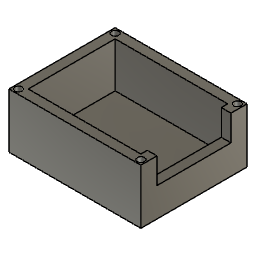
Bottom Battery Holder v2 (Autodesk Fusion 360 design; units mm, degrees)
Autodesk Fusion 360 part; units mm, degrees
(part 1 of 2)
sketch "Sketch1" plane through (0, 0, 0) normal (0, 0, 1) x (1, 0, 0)
  line L0 (0, 0) -> (41, 0)
  line L1 (41, 0) -> (41, 33)
  line L2 (41, 33) -> (0, 33)
  line L3 (0, 33) -> (0, 0)
  dimension "d1" = 41
  dimension "d2" = 33
  constraint horizontal L0
  constraint vertical L1
  constraint horizontal L2
  constraint vertical L3
  constraint coincident L0.start L3.end
  measures "d1" distance of L0.start L0.end
  measures "d2" distance of L0.start L2.end
extrude "Extrude1" add sketch "Sketch1" along normal blind 17
sketch "Sketch2" plane through (0, 0, 17) normal (0, 0, 1) x (-1, 0, 0)
  line L0 (0, -33) -> (0, 0)
  line L1 (0, 0) -> (-41, 0)
  line L2 (-41, 0) -> (-41, -33)
  line L3 (-41, -33) -> (0, -33)
  line L4 (-3, -3) -> (-38, -3)
  line L5 (-38, -3) -> (-38, -30)
  line L6 (-38, -30) -> (-3, -30)
  line L7 (-3, -30) -> (-3, -3)
  dimension "d5" = 35
  dimension "d6" = 27
  constraint horizontal L4
  constraint vertical L5
  constraint horizontal L6
  constraint vertical L7
  measures "d5" distance of L4.start L4.end
  measures "d6" distance of L4.start L6.end
extrude "Extrude2" cut sketch "Sketch2" against normal blind 14 contours L4 L5 L6 L7
sketch "Sketch3" plane through (41, 0, 0) normal (1, 0, 0) x (0, 1, 0)
  line L0 (0, 0) -> (33, 0)
  line L1 (33, 0) -> (33, 17)
  line L2 (33, 17) -> (0, 17)
  line L3 (0, 17) -> (0, 0)
  line L4 (4.9994, 17) -> (28, 17)
  line L5 (28, 17) -> (28, 9)
  line L6 (28, 9) -> (4.9994, 9)
  line L7 (4.9994, 9) -> (4.9994, 17)
  constraint horizontal L4
  constraint vertical L5
  constraint horizontal L6
  constraint vertical L7
  constraint coincident L2 L4.start
extrude "Extrude3" cut sketch "Sketch3" against normal blind 10 contours L2 L4 L5 L6 L7
sketch "Sketch4" plane through (0, 0, 17) normal (0, 0, 1) x (-1, 0, 0)
  line L0 (-41, -4.9994) -> (-38, -4.9994)
  line L1 (-38, -4.9994) -> (-38, -3)
  line L2 (-38, -3) -> (-3, -3)
  line L3 (-3, -3) -> (-3, -30)
  line L4 (-3, -30) -> (-38, -30)
  line L5 (-38, -30) -> (-38, -28)
  line L6 (-38, -28) -> (-41, -28)
  line L7 (-41, -28) -> (-41, -33)
  line L8 (-41, -33) -> (0, -33)
  line L9 (0, -33) -> (0, 0)
  line L10 (0, 0) -> (-41, 0)
  line L11 (-41, 0) -> (-41, -4.9994)
  circle A0 centre (-1.5, -31.5) radius 1.118
  circle A1 centre (-1.5, -1.4974) radius 1.1192
  circle A2 centre (-39.5, -1.5) radius 1.118
  circle A3 centre (-39.5, -31.5) radius 1.118
  dimension "d11" = 2.2384
  dimension "d12" = 2.2361
  dimension "d13" = 2.236
  measures "d11" diameter of A1
  measures "d12" diameter of A0
  measures "d13" diameter of A3
extrude "Extrude4" cut sketch "Sketch4" against normal blind 10 contours A0 | A1 | A2 | A3
sketch "falmouthrobotics" plane through (0, 0, 0) normal (0, 0, -1) x (-1, 0, 0)
  arc A0 through (-5.6563, 11.59, -1.2301) (-5.3945, 11.4792, -1.2301) (-5.1327, 11.3684, -1.2301)
  arc A1 through (-5.1327, 11.3684, -1.2301) (-5.117, 11.3607, -1.2301) (-5.1022, 11.3515, -1.2301)
  arc A2 through (-32.1117, 13.7154, -1.2301) (-32.0879, 13.6563, -1.2301) (-32.0476, 13.607, -1.2301)
  arc A3 through (-15.3811, 14.3738, -1.2301) (-15.4462, 14.3529, -1.2301) (-15.5092, 14.3263, -1.2301)
  line L0 (-34.3881, 15.5149, -1.2301) -> (-33.2917, 15.5149, -1.2301)
  arc A4 through (-8.6784, 13.2928, -1.2301) (-8.7193, 13.2009, -1.2301) (-8.7575, 13.1079, -1.2301)
  arc A5 through (-7.6435, 12.4319, -1.2301) (-7.2917, 12.278, -1.2301) (-6.9381, 12.1281, -1.2301)
  arc A6 through (-5.1022, 11.3515, -1.2301) (-5.0953, 11.3416, -1.2301) (-5.0965, 11.3296, -1.2301)
  arc A7 through (-5.1403, 11.2447, -1.2301) (-5.1702, 11.1924, -1.2301) (-5.2021, 11.1412, -1.2301)
  arc A8 through (-15.5881, 14.2649, -1.2301) (-15.6327, 14.1862, -1.2301) (-15.6472, 14.0969, -1.2301)
  line L1 (-34.3881, 14.6527, -1.2301) -> (-34.3881, 15.5149, -1.2301)
  arc A9 through (-33.2653, 15.9925, -1.2301) (-33.6488, 15.998, -1.2301) (-34.0323, 16.0007, -1.2301)
  line L2 (-32.1954, 15.5149, -1.2301) -> (-32.1667, 14.5399, -1.2301)
  arc A10 through (-14.5007, 14.281, -1.2301) (-14.6017, 14.3449, -1.2301) (-14.7151, 14.3826, -1.2301)
  arc A11 through (-6.2455, 11.8382, -1.2301) (-5.9508, 11.7143, -1.2301) (-5.6563, 11.59, -1.2301)
  arc A12 through (-8.7575, 13.1079, -1.2301) (-8.7675, 13.0656, -1.2301) (-8.7654, 13.0223, -1.2301)
  arc A13 through (-32.1444, 13.9508, -1.2301) (-32.1335, 13.8323, -1.2301) (-32.1117, 13.7154, -1.2301)
  line L3 (-32.7772, 12.1034, -1.2301) -> (-34.3881, 13.7905, -1.2301)
  arc A14 through (-4.5188, 11.422, -1.2301) (-4.5087, 11.4642, -1.2301) (-4.5108, 11.5076, -1.2301)
  line L4 (-6.7536, 14.2928, -1.2301) -> (-8.0692, 14.3206, -1.2301)
  line L5 (-7.9945, 13.506, -1.2301) -> (-7.779, 13.8087, -1.2301)
  arc A15 through (-8.7654, 13.0223, -1.2301) (-8.745, 12.9761, -1.2301) (-8.7064, 12.9436, -1.2301)
  arc A16 through (-8.5827, 10.2892, -1.2301) (-8.3781, 10.2689, -1.2301) (-8.1726, 10.2591, -1.2301)
  line L6 (-30.4381, 10.1649, -1.2301) -> (-28.9381, 10.1649, -1.2301)
  arc A17 through (-4.5977, 11.2373, -1.2301) (-4.5568, 11.329, -1.2301) (-4.5188, 11.422, -1.2301)
  line L7 (-28.9381, 10.1649, -1.2301) -> (-27.4381, 10.1649, -1.2301)
  arc A18 through (-5.4381, 14.0649, -1.2301) (-5.4521, 14.1267, -1.2301) (-5.4914, 14.1764, -1.2301)
  arc A19 through (-14.7151, 14.3826, -1.2301) (-14.8758, 14.4068, -1.2301) (-15.0381, 14.4149, -1.2301)
  arc A20 through (-8.1361, 13.2849, -1.2301) (-8.1062, 13.3371, -1.2301) (-8.0745, 13.3882, -1.2301)
  line L8 (-34.3381, 13.0329, -1.2301) -> (-32.9548, 11.5739, -1.2301)
  arc A21 through (-28.9152, 14.0926, -1.2301) (-29.2888, 14.0982, -1.2301) (-29.6625, 14.1009, -1.2301)
  arc A22 through (-8.1436, 13.1615, -1.2301) (-8.1592, 13.1691, -1.2301) (-8.174, 13.1783, -1.2301)
  arc A23 through (-29.6625, 14.1009, -1.2301) (-29.8782, 14.0978, -1.2301) (-30.0937, 14.0871, -1.2301)
  arc A24 through (-8.601, 10.6404, -1.2301) (-8.691, 10.6185, -1.2301) (-8.7746, 10.5784, -1.2301)
  arc A25 through (-7.0308, 12.6917, -1.2301) (-7.3254, 12.8156, -1.2301) (-7.6199, 12.9399, -1.2301)
  arc A26 through (-31.9381, 13.5649, -1.2301) (-31.8778, 13.5777, -1.2301) (-31.828, 13.614, -1.2301)
  arc A27 through (-7.1682, 10.6923, -1.2301) (-7.6947, 10.6826, -1.2301) (-8.2211, 10.6708, -1.2301)
  line L9 (-31.7381, 14.7649, -1.2301) -> (-31.7381, 15.9649, -1.2301)
  arc A28 through (-31.5196, 10.1515, -1.2301) (-31.4766, 10.1244, -1.2301) (-31.4267, 10.1149, -1.2301)
  arc A29 through (-15.5756, 13.9489, -1.2301) (-15.4746, 13.885, -1.2301) (-15.3612, 13.8472, -1.2301)
  arc A30 through (-8.7064, 12.9436, -1.2301) (-8.4675, 12.8229, -1.2301) (-8.2277, 12.7043, -1.2301)
  arc A31 through (-5.0965, 11.3296, -1.2301) (-5.1179, 11.2869, -1.2301) (-5.1403, 11.2447, -1.2301)
  arc A32 through (-34.7609, 15.9565, -1.2301) (-34.8102, 15.9347, -1.2301) (-34.8419, 15.8912, -1.2301)
  arc A33 through (-31.7673, 13.7399, -1.2301) (-31.7496, 13.8786, -1.2301) (-31.7426, 14.0182, -1.2301)
  line L10 (-31.7381, 15.9649, -1.2301) -> (-33.2653, 15.9925, -1.2301)
  arc A34 through (-15.5092, 14.3263, -1.2301) (-15.552, 14.2999, -1.2301) (-15.5881, 14.2649, -1.2301)
  arc A35 through (-5.2021, 11.1412, -1.2301) (-5.2415, 11.0817, -1.2301) (-5.2823, 11.0231, -1.2301)
  arc A36 through (-34.0323, 16.0007, -1.2301) (-34.2562, 15.9976, -1.2301) (-34.4798, 15.987, -1.2301)
  arc A37 through (-8.5675, 13.511, -1.2301) (-8.6249, 13.4029, -1.2301) (-8.6784, 13.2928, -1.2301)
  line L11 (-34.3881, 13.7905, -1.2301) -> (-34.3881, 14.6527, -1.2301)
  line L12 (-5.2823, 11.0231, -1.2301) -> (-5.4983, 10.7197, -1.2301)
  arc A38 through (-15.6472, 14.0969, -1.2301) (-15.6277, 14.015, -1.2301) (-15.5756, 13.9489, -1.2301)
  arc A39 through (-8.2277, 12.7043, -1.2301) (-7.9369, 12.5653, -1.2301) (-7.6435, 12.4319, -1.2301)
  arc A40 through (-32.1667, 14.5399, -1.2301) (-32.1568, 14.2453, -1.2301) (-32.1444, 13.9508, -1.2301)
  line L13 (-5.4983, 10.7197, -1.2301) -> (-7.1682, 10.6923, -1.2301)
  arc A41 through (-31.9353, 10.5435, -1.2301) (-31.7281, 10.3469, -1.2301) (-31.5196, 10.1515, -1.2301)
  arc A42 through (-31.2884, 10.2421, -1.2301) (-31.3002, 10.3789, -1.2301) (-31.357, 10.5039, -1.2301)
  arc A43 through (-31.828, 13.614, -1.2301) (-31.7886, 13.6726, -1.2301) (-31.7673, 13.7399, -1.2301)
  arc A44 through (-14.4881, 13.9649, -1.2301) (-14.4435, 14.0437, -1.2301) (-14.429, 14.133, -1.2301)
  arc A45 through (-8.4309, 13.7428, -1.2301) (-8.5008, 13.6278, -1.2301) (-8.5675, 13.511, -1.2301)
  arc A46 through (-31.4267, 10.1149, -1.2301) (-31.3327, 10.1516, -1.2301) (-31.2884, 10.2421, -1.2301)
  arc A47 through (-15.0381, 13.8149, -1.2301) (-14.947, 13.8175, -1.2301) (-14.8563, 13.8252, -1.2301)
  arc A48 through (-32.0476, 13.607, -1.2301) (-31.9968, 13.5758, -1.2301) (-31.9381, 13.5649, -1.2301)
  arc A49 through (-30.4723, 12.7289, -1.2301) (-30.4698, 12.3703, -1.2301) (-30.4655, 12.0117, -1.2301)
  line L14 (-33.2917, 15.5149, -1.2301) -> (-32.1954, 15.5149, -1.2301)
  arc A50 through (-32.4141, 11.0147, -1.2301) (-32.1765, 10.7773, -1.2301) (-31.9353, 10.5435, -1.2301)
  arc A51 through (-5.0486, 11.8256, -1.2301) (-5.3394, 11.9645, -1.2301) (-5.6327, 12.098, -1.2301)
  arc A52 through (-7.6199, 12.9399, -1.2301) (-7.8818, 13.0507, -1.2301) (-8.1436, 13.1615, -1.2301)
  arc A53 through (-4.8449, 10.7877, -1.2301) (-4.7752, 10.9025, -1.2301) (-4.7085, 11.0192, -1.2301)
  arc A54 through (-30.47, 13.3545, -1.2301) (-30.4724, 13.0417, -1.2301) (-30.4723, 12.7289, -1.2301)
  arc A55 through (-5.4914, 14.1764, -1.2301) (-5.5572, 14.217, -1.2301) (-5.631, 14.2397, -1.2301)
  line L15 (-27.4381, 14.0649, -1.2301) -> (-28.9152, 14.0926, -1.2301)
  line L16 (-5.2063, 10.2105, -1.2301) -> (-4.8449, 10.7877, -1.2301)
  arc A56 through (-4.5108, 11.5076, -1.2301) (-4.5313, 11.5538, -1.2301) (-4.5699, 11.5863, -1.2301)
  arc A57 through (-4.7085, 11.0192, -1.2301) (-4.6512, 11.1272, -1.2301) (-4.5977, 11.2373, -1.2301)
  arc A58 through (-5.6327, 12.098, -1.2301) (-5.9846, 12.2518, -1.2301) (-6.3381, 12.4017, -1.2301)
  arc A59 through (-8.0745, 13.3882, -1.2301) (-8.0351, 13.4476, -1.2301) (-7.9945, 13.506, -1.2301)
  line L17 (-7.779, 13.8087, -1.2301) -> (-6.6085, 13.8368, -1.2301)
  line L18 (-8.0692, 14.3206, -1.2301) -> (-8.4309, 13.7428, -1.2301)
  arc A60 through (-8.7746, 10.5784, -1.2301) (-8.8212, 10.53, -1.2301) (-8.8381, 10.4649, -1.2301)
  arc A61 through (-5.631, 14.2397, -1.2301) (-5.7836, 14.2607, -1.2301) (-5.9373, 14.271, -1.2301)
  arc A62 through (-5.9373, 14.271, -1.2301) (-6.3454, 14.283, -1.2301) (-6.7536, 14.2928, -1.2301)
  arc A63 through (-8.8381, 10.4649, -1.2301) (-8.8201, 10.3986, -1.2301) (-8.7708, 10.3506, -1.2301)
  line L19 (-27.4381, 10.1649, -1.2301) -> (-27.4381, 12.1149, -1.2301)
  arc A64 through (-8.174, 13.1783, -1.2301) (-8.1809, 13.1882, -1.2301) (-8.1798, 13.2002, -1.2301)
  arc A65 through (-8.1726, 10.2591, -1.2301) (-7.5974, 10.2474, -1.2301) (-7.0222, 10.2377, -1.2301)
  line L20 (-30.4655, 12.0117, -1.2301) -> (-30.4381, 10.1649, -1.2301)
  arc A66 through (-5.4868, 13.9542, -1.2301) (-5.4508, 14.0045, -1.2301) (-5.4381, 14.0649, -1.2301)
  arc A67 through (-8.1798, 13.2002, -1.2301) (-8.1585, 13.2429, -1.2301) (-8.1361, 13.2849, -1.2301)
  arc A68 through (-30.4621, 13.8893, -1.2301) (-30.4665, 13.6219, -1.2301) (-30.47, 13.3545, -1.2301)
  arc A69 through (-4.5699, 11.5863, -1.2301) (-4.8087, 11.7069, -1.2301) (-5.0486, 11.8256, -1.2301)
  line L21 (-27.4381, 12.1149, -1.2301) -> (-27.4381, 14.0649, -1.2301)
  arc A70 through (-8.7708, 10.3506, -1.2301) (-8.6797, 10.3109, -1.2301) (-8.5827, 10.2892, -1.2301)
  arc A71 through (-6.3381, 12.4017, -1.2301) (-6.6845, 12.5466, -1.2301) (-7.0308, 12.6917, -1.2301)
  line L22 (-7.0222, 10.2377, -1.2301) -> (-5.2063, 10.2105, -1.2301)
  arc A72 through (-6.6085, 13.8368, -1.2301) (-6.2487, 13.8466, -1.2301) (-5.889, 13.8588, -1.2301)
  arc A73 through (-5.889, 13.8588, -1.2301) (-5.7504, 13.8693, -1.2301) (-5.6129, 13.8906, -1.2301)
  arc A74 through (-30.4426, 13.9894, -1.2301) (-30.4567, 13.9402, -1.2301) (-30.4621, 13.8893, -1.2301)
  arc A75 through (-8.2211, 10.6708, -1.2301) (-8.4115, 10.6609, -1.2301) (-8.601, 10.6404, -1.2301)
  arc A76 through (-5.6129, 13.8906, -1.2301) (-5.5455, 13.9137, -1.2301) (-5.4868, 13.9542, -1.2301)
  arc A77 through (-22.3721, 21.0063, -1.2301) (-22.5314, 21.0347, -1.2301) (-22.6925, 21.0501, -1.2301)
  arc A78 through (-20.2423, 17.2748, -1.2301) (-20.1749, 17.3588, -1.2301) (-20.1417, 17.4613, -1.2301)
  arc A79 through (-20.123, 17.9253, -1.2301) (-20.1529, 18.4515, -1.2301) (-20.1882, 18.9774, -1.2301)
  arc A80 through (-20.8687, 20.3549, -1.2301) (-20.7876, 20.1081, -1.2301) (-20.7457, 19.8517, -1.2301)
  arc A81 through (-31.3022, 19.6901, -1.2301) (-31.4368, 19.2445, -1.2301) (-31.5647, 18.7969, -1.2301)
  arc A82 through (-31.1005, 17.5695, -1.2301) (-30.9592, 17.5368, -1.2301) (-30.8157, 17.515, -1.2301)
  arc A83 through (-29.6034, 17.4414, -1.2301) (-29.4771, 17.4467, -1.2301) (-29.3512, 17.4562, -1.2301)
  arc A84 through (-23.9816, 21.4831, -1.2301) (-24.047, 21.5096, -1.2301) (-24.1176, 21.5076, -1.2301)
  line L23 (-30.5878, 20.6825, -1.2301) -> (-31.0375, 20.543, -1.2301)
  arc A85 through (-20.7284, 20.9621, -1.2301) (-20.847, 21.0193, -1.2301) (-20.974, 21.054, -1.2301)
  arc A86 through (-30.3134, 17.4669, -1.2301) (-30.1203, 17.4535, -1.2301) (-29.9269, 17.4438, -1.2301)
  arc A87 through (-28.7881, 20.9358, -1.2301) (-28.7899, 20.8267, -1.2301) (-28.7952, 20.7177, -1.2301)
  arc A88 through (-20.974, 21.054, -1.2301) (-21.1103, 21.0662, -1.2301) (-21.2466, 21.0547, -1.2301)
  arc A89 through (-24.1176, 21.5076, -1.2301) (-24.183, 21.4775, -1.2301) (-24.232, 21.4248, -1.2301)
  arc A90 through (-23.7217, 20.819, -1.2301) (-23.7327, 20.8159, -1.2301) (-23.744, 20.8149, -1.2301)
  arc A91 through (-20.4913, 17.3172, -1.2301) (-20.4631, 17.2726, -1.2301) (-20.4189, 17.2437, -1.2301)
  arc A92 through (-28.7832, 21.0731, -1.2301) (-28.7869, 21.0045, -1.2301) (-28.7881, 20.9358, -1.2301)
  arc A93 through (-20.5898, 17.8097, -1.2301) (-20.5714, 17.6585, -1.2301) (-20.5452, 17.5083, -1.2301)
  arc A94 through (-28.7952, 20.7177, -1.2301) (-28.806, 20.6779, -1.2301) (-28.8315, 20.6455, -1.2301)
  arc A95 through (-30.2665, 20.7566, -1.2301) (-30.4285, 20.7255, -1.2301) (-30.5878, 20.6825, -1.2301)
  arc A96 through (-29.9269, 17.4438, -1.2301) (-29.7652, 17.4399, -1.2301) (-29.6034, 17.4414, -1.2301)
  arc A97 through (-23.7754, 20.9102, -1.2301) (-23.7847, 20.9624, -1.2301) (-23.7925, 21.0148, -1.2301)
  arc A98 through (-20.7457, 19.8517, -1.2301) (-20.6831, 19.0671, -1.2301) (-20.6278, 18.282, -1.2301)
  arc A99 through (-23.7925, 21.0148, -1.2301) (-23.8002, 21.0769, -1.2301) (-23.8068, 21.1391, -1.2301)
  arc A100 through (-21.5495, 20.9666, -1.2301) (-21.6891, 20.9127, -1.2301) (-21.8313, 20.8664, -1.2301)
  arc A101 through (-23.3635, 20.9608, -1.2301) (-23.4314, 20.9326, -1.2301) (-23.4995, 20.9049, -1.2301)
  arc A102 through (-22.07, 20.8212, -1.2301) (-22.1517, 20.8204, -1.2301) (-22.2326, 20.8323, -1.2301)
  arc A103 through (-28.7215, 21.3483, -1.2301) (-28.7375, 21.3271, -1.2301) (-28.7474, 21.3024, -1.2301)
  arc A104 through (-20.4189, 17.2437, -1.2301) (-20.3263, 17.2348, -1.2301) (-20.2423, 17.2748, -1.2301)
  arc A105 through (-31.6486, 18.3294, -1.2301) (-31.6462, 18.176, -1.2301) (-31.6134, 18.0261, -1.2301)
  arc A106 through (-23.7576, 20.8258, -1.2301) (-23.7669, 20.8679, -1.2301) (-23.7754, 20.9102, -1.2301)
  arc A107 through (-23.8068, 21.1391, -1.2301) (-23.8262, 21.2445, -1.2301) (-23.8633, 21.3451, -1.2301)
  arc A108 through (-28.7474, 21.3024, -1.2301) (-28.7591, 21.2512, -1.2301) (-28.7685, 21.1996, -1.2301)
  arc A109 through (-31.4628, 17.7805, -1.2301) (-31.383, 17.7104, -1.2301) (-31.2949, 17.6511, -1.2301)
  arc A110 through (-23.0627, 21.0391, -1.2301) (-23.2159, 21.0106, -1.2301) (-23.3635, 20.9608, -1.2301)
  arc A111 through (-22.2881, 20.9018, -1.2301) (-22.3117, 20.9689, -1.2301) (-22.3721, 21.0063, -1.2301)
  arc A112 through (-22.6925, 21.0501, -1.2301) (-22.8778, 21.0524, -1.2301) (-23.0627, 21.0391, -1.2301)
  arc A113 through (-21.1031, 20.5148, -1.2301) (-20.9622, 20.4696, -1.2301) (-20.8687, 20.3549, -1.2301)
  line L24 (-31.0375, 20.543, -1.2301) -> (-31.3022, 19.6901, -1.2301)
  arc A114 through (-20.6278, 18.282, -1.2301) (-20.6105, 18.0457, -1.2301) (-20.5898, 17.8097, -1.2301)
  arc A115 through (-28.8315, 20.6455, -1.2301) (-28.8672, 20.6264, -1.2301) (-28.9076, 20.6235, -1.2301)
  arc A116 through (-23.4995, 20.9049, -1.2301) (-23.5593, 20.8811, -1.2301) (-23.6192, 20.8578, -1.2301)
  arc A117 through (-30.8157, 17.515, -1.2301) (-30.5648, 17.4889, -1.2301) (-30.3134, 17.4669, -1.2301)
  arc A118 through (-31.5647, 18.7969, -1.2301) (-31.6176, 18.5651, -1.2301) (-31.6486, 18.3294, -1.2301)
  arc A119 through (-22.2326, 20.8323, -1.2301) (-22.2726, 20.8574, -1.2301) (-22.2881, 20.9018, -1.2301)
  arc A120 through (-28.7685, 21.1996, -1.2301) (-28.7773, 21.1365, -1.2301) (-28.7832, 21.0731, -1.2301)
  arc A121 through (-29.1131, 20.6602, -1.2301) (-29.3497, 20.7076, -1.2301) (-29.5876, 20.7478, -1.2301)
  arc A122 through (-23.6192, 20.8578, -1.2301) (-23.6705, 20.8383, -1.2301) (-23.7217, 20.819, -1.2301)
  arc A123 through (-20.5052, 20.7815, -1.2301) (-20.6105, 20.8796, -1.2301) (-20.7284, 20.9621, -1.2301)
  arc A124 through (-30.8792, 19.373, -1.2301) (-30.8186, 19.5693, -1.2301) (-30.7537, 19.7643, -1.2301)
  arc A125 through (-16.5788, 20.6817, -1.2301) (-16.812, 20.9833, -1.2301) (-17.1105, 21.2203, -1.2301)
  line L25 (-29.1664, 18.224, -1.2301) -> (-29.4448, 17.8906, -1.2301)
  arc A126 through (-17.756, 21.3925, -1.2301) (-18.0918, 21.3348, -1.2301) (-18.3983, 21.1861, -1.2301)
  arc A127 through (-30.5432, 20.1183, -1.2301) (-30.4753, 20.1673, -1.2301) (-30.3997, 20.2032, -1.2301)
  arc A128 through (-18.3983, 21.1861, -1.2301) (-18.5943, 21.0334, -1.2301) (-18.7674, 20.8551, -1.2301)
  arc A129 through (-29.9842, 20.2998, -1.2301) (-29.8802, 20.2943, -1.2301) (-29.7772, 20.2791, -1.2301)
  arc A130 through (-28.4107, 21.3813, -1.2301) (-28.4635, 21.4015, -1.2301) (-28.5191, 21.4116, -1.2301)
  arc A131 through (-17.1105, 21.2203, -1.2301) (-17.4207, 21.3535, -1.2301) (-17.756, 21.3925, -1.2301)
  arc A132 through (-30.6529, 19.9851, -1.2301) (-30.6036, 20.0562, -1.2301) (-30.5432, 20.1183, -1.2301)
  arc A133 through (-31.0392, 18.7702, -1.2301) (-31.0028, 18.9208, -1.2301) (-30.9642, 19.0709, -1.2301)
  line L26 (-29.3958, 20.1978, -1.2301) -> (-28.8881, 20.0806, -1.2301)
  arc A134 through (-17.0441, 20.5977, -1.2301) (-16.9073, 20.2808, -1.2301) (-16.8044, 19.9512, -1.2301)
  arc A135 through (-16.6982, 19.2296, -1.2301) (-16.7154, 18.9391, -1.2301) (-16.7907, 18.6581, -1.2301)
  arc A136 through (-28.6332, 21.4004, -1.2301) (-28.6806, 21.3799, -1.2301) (-28.7215, 21.3483, -1.2301)
  arc A137 through (-16.7907, 18.6581, -1.2301) (-16.8246, 18.6038, -1.2301) (-16.8767, 18.5666, -1.2301)
  arc A138 through (-16.8767, 18.5666, -1.2301) (-16.9295, 18.5608, -1.2301) (-16.9754, 18.5876, -1.2301)
  arc A139 through (-28.9332, 18.6267, -1.2301) (-28.966, 18.5292, -1.2301) (-29.013, 18.4377, -1.2301)
  arc A140 through (-19.2381, 19.3149, -1.2301) (-19.2251, 19.0086, -1.2301) (-19.1863, 18.7044, -1.2301)
  arc A141 through (-19.0304, 18.1925, -1.2301) (-18.9135, 17.9744, -1.2301) (-18.7674, 17.7747, -1.2301)
  arc A142 through (-29.1389, 17.5313, -1.2301) (-29.0952, 17.5399, -1.2301) (-29.0508, 17.5418, -1.2301)
  arc A143 through (-23.8633, 21.3451, -1.2301) (-23.9131, 21.4222, -1.2301) (-23.9816, 21.4831, -1.2301)
  arc A144 through (-17.366, 20.9095, -1.2301) (-17.1782, 20.7814, -1.2301) (-17.0441, 20.5977, -1.2301)
  arc A145 through (-19.1863, 19.9254, -1.2301) (-19.2251, 19.6213, -1.2301) (-19.2381, 19.3149, -1.2301)
  line L27 (-30.2914, 17.9778, -1.2301) -> (-31.1381, 18.0649, -1.2301)
  arc A146 through (-31.2949, 17.6511, -1.2301) (-31.2004, 17.6039, -1.2301) (-31.1005, 17.5695, -1.2301)
  arc A147 through (-31.6134, 18.0261, -1.2301) (-31.5526, 17.8944, -1.2301) (-31.4628, 17.7805, -1.2301)
  arc A148 through (-20.1882, 18.9774, -1.2301) (-20.2219, 19.4191, -1.2301) (-20.2587, 19.8606, -1.2301)
  arc A149 through (-20.2587, 19.8606, -1.2301) (-20.2838, 20.0905, -1.2301) (-20.3188, 20.319, -1.2301)
  arc A150 through (-28.8973, 18.8727, -1.2301) (-28.9088, 18.7488, -1.2301) (-28.9332, 18.6267, -1.2301)
  arc A151 through (-28.9624, 17.5251, -1.2301) (-28.9161, 17.5059, -1.2301) (-28.8721, 17.4817, -1.2301)
  arc A152 through (-28.9076, 20.6235, -1.2301) (-29.0107, 20.64, -1.2301) (-29.1131, 20.6602, -1.2301)
  arc A153 through (-18.7674, 20.8551, -1.2301) (-18.9135, 20.6555, -1.2301) (-19.0304, 20.4374, -1.2301)
  arc A154 through (-19.0304, 20.4374, -1.2301) (-19.1245, 20.1863, -1.2301) (-19.1863, 19.9254, -1.2301)
  arc A155 through (-28.65, 17.4333, -1.2301) (-28.6216, 17.4474, -1.2301) (-28.597, 17.4674, -1.2301)
  arc A156 through (-28.3385, 21.3155, -1.2301) (-28.37, 21.3534, -1.2301) (-28.4107, 21.3813, -1.2301)
  arc A157 through (-29.013, 18.4377, -1.2301) (-29.0858, 18.3281, -1.2301) (-29.1664, 18.224, -1.2301)
  line L28 (-31.1381, 18.0649, -1.2301) -> (-31.1177, 18.3519, -1.2301)
  arc A158 through (-18.3983, 17.4438, -1.2301) (-17.9918, 17.2721, -1.2301) (-17.5505, 17.2664, -1.2301)
  arc A159 through (-29.3512, 17.4562, -1.2301) (-29.2878, 17.4688, -1.2301) (-29.2285, 17.4943, -1.2301)
  arc A160 through (-29.0508, 17.5418, -1.2301) (-29.0059, 17.5368, -1.2301) (-28.9624, 17.5251, -1.2301)
  arc A161 through (-29.7772, 20.2791, -1.2301) (-29.5862, 20.24, -1.2301) (-29.3958, 20.1978, -1.2301)
  arc A162 through (-28.5191, 21.4116, -1.2301) (-28.5767, 21.4112, -1.2301) (-28.6332, 21.4004, -1.2301)
  arc A163 through (-30.3997, 20.2032, -1.2301) (-30.2813, 20.2433, -1.2301) (-30.1611, 20.2777, -1.2301)
  line L29 (-29.4448, 17.8906, -1.2301) -> (-30.2914, 17.9778, -1.2301)
  arc A164 through (-18.7674, 17.7747, -1.2301) (-18.5943, 17.5965, -1.2301) (-18.3983, 17.4438, -1.2301)
  arc A165 through (-28.7144, 17.4236, -1.2301) (-28.6817, 17.4252, -1.2301) (-28.65, 17.4333, -1.2301)
  arc A166 through (-28.5117, 17.6556, -1.2301) (-28.4505, 18.5163, -1.2301) (-28.3915, 19.3771, -1.2301)
  arc A167 through (-16.2647, 19.8768, -1.2301) (-16.3884, 20.2923, -1.2301) (-16.5788, 20.6817, -1.2301)
  arc A168 through (-30.9642, 19.0709, -1.2301) (-30.9228, 19.2222, -1.2301) (-30.8792, 19.373, -1.2301)
  arc A169 through (-19.1863, 18.7044, -1.2301) (-19.1245, 18.4435, -1.2301) (-19.0304, 18.1925, -1.2301)
  arc A170 through (-31.1177, 18.3519, -1.2301) (-31.1095, 18.4304, -1.2301) (-31.0963, 18.5083, -1.2301)
  arc A171 through (-28.3915, 19.3771, -1.2301) (-28.3353, 20.2331, -1.2301) (-28.2816, 21.0891, -1.2301)
  arc A172 through (-28.2816, 21.0891, -1.2301) (-28.2925, 21.2067, -1.2301) (-28.3385, 21.3155, -1.2301)
  arc A173 through (-16.7549, 17.7173, -1.2301) (-16.4469, 18.1754, -1.2301) (-16.2651, 18.6966, -1.2301)
  arc A174 through (-26.6603, 16.0898, -1.2301) (-26.6646, 15.6627, -1.2301) (-26.6684, 15.2356, -1.2301)
  arc A175 through (-30.1611, 20.2777, -1.2301) (-30.0734, 20.2945, -1.2301) (-29.9842, 20.2998, -1.2301)
  line L30 (-26.1881, 10.6149, -1.2301) -> (-26.1881, 11.6149, -1.2301)
  arc A176 through (-26.316, 16.2157, -1.2301) (-26.3545, 16.2683, -1.2301) (-26.4134, 16.2961, -1.2301)
  line L31 (-24.3881, 10.6149, -1.2301) -> (-25.2881, 10.6149, -1.2301)
  arc A177 through (-34.8419, 15.8912, -1.2301) (-34.8562, 15.8408, -1.2301) (-34.8615, 15.7886, -1.2301)
  arc A178 through (-17.2745, 17.697, -1.2301) (-17.3839, 17.6601, -1.2301) (-17.4974, 17.6387, -1.2301)
  arc A179 through (-26.2316, 15.6099, -1.2301) (-26.2422, 15.81, -1.2301) (-26.2625, 16.0094, -1.2301)
  arc A180 through (-18.5686, 18.3959, -1.2301) (-18.6408, 18.6293, -1.2301) (-18.6957, 18.8673, -1.2301)
  arc A181 through (-17.2224, 17.7885, -1.2301) (-17.2328, 17.7338, -1.2301) (-17.2745, 17.697, -1.2301)
  line L32 (-25.2881, 12.6149, -1.2301) -> (-24.3881, 12.6149, -1.2301)
  arc A182 through (-34.8147, 10.5431, -1.2301) (-34.7943, 10.396, -1.2301) (-34.7575, 10.2522, -1.2301)
  arc A183 through (-26.6711, 14.2537, -1.2301) (-26.6689, 13.6837, -1.2301) (-26.6647, 13.1138, -1.2301)
  arc A184 through (-16.9754, 18.5876, -1.2301) (-17.0617, 18.6944, -1.2301) (-17.1381, 18.8084, -1.2301)
  line L33 (-28.8881, 20.0806, -1.2301) -> (-28.8881, 19.319, -1.2301)
  arc A185 through (-17.4974, 17.6387, -1.2301) (-17.6335, 17.6284, -1.2301) (-17.77, 17.6295, -1.2301)
  arc A186 through (-18.0833, 20.4151, -1.2301) (-18.1786, 20.5872, -1.2301) (-18.2734, 20.7596, -1.2301)
  line L34 (-24.3881, 12.6149, -1.2301) -> (-24.3881, 11.6149, -1.2301)
  arc A187 through (-18.2881, 20.8172, -1.2301) (-18.2661, 20.8889, -1.2301) (-18.2076, 20.9359, -1.2301)
  arc A188 through (-17.9589, 20.9967, -1.2301) (-17.8025, 21.003, -1.2301) (-17.6463, 20.9908, -1.2301)
  arc A189 through (-34.869, 14.978, -1.2301) (-34.8714, 14.5118, -1.2301) (-34.8714, 14.0456, -1.2301)
  arc A190 through (-31.0963, 18.5083, -1.2301) (-31.0687, 18.6394, -1.2301) (-31.0392, 18.7702, -1.2301)
  arc A191 through (-17.5505, 17.2664, -1.2301) (-17.1145, 17.4245, -1.2301) (-16.7549, 17.7173, -1.2301)
  arc A192 through (-28.8881, 19.319, -1.2301) (-28.8904, 19.0958, -1.2301) (-28.8973, 18.8727, -1.2301)
  line L35 (-24.3881, 11.6149, -1.2301) -> (-24.3881, 10.6149, -1.2301)
  arc A193 through (-29.2285, 17.4943, -1.2301) (-29.1848, 17.5155, -1.2301) (-29.1389, 17.5313, -1.2301)
  arc A194 through (-28.8721, 17.4817, -1.2301) (-28.8316, 17.4589, -1.2301) (-28.7891, 17.4399, -1.2301)
  line L36 (-26.6647, 13.1138, -1.2301) -> (-26.6381, 10.1649, -1.2301)
  arc A195 through (-17.858, 20.018, -1.2301) (-17.9715, 20.2161, -1.2301) (-18.0833, 20.4151, -1.2301)
  arc A196 through (-18.6957, 18.8673, -1.2301) (-18.7275, 19.0885, -1.2301) (-18.7381, 19.3117, -1.2301)
  arc A197 through (-34.4601, 10.3754, -1.2301) (-34.4366, 10.5419, -1.2301) (-34.4237, 10.7094, -1.2301)
  arc A198 through (-18.3985, 19.9244, -1.2301) (-18.1196, 19.468, -1.2301) (-17.8453, 19.0089, -1.2301)
  arc A199 through (-30.7537, 19.7643, -1.2301) (-30.7086, 19.8771, -1.2301) (-30.6529, 19.9851, -1.2301)
  arc A200 through (-17.4496, 18.3268, -1.2301) (-17.359, 18.1573, -1.2301) (-17.2776, 17.9833, -1.2301)
  arc A201 through (-18.2076, 20.9359, -1.2301) (-18.0854, 20.975, -1.2301) (-17.9589, 20.9967, -1.2301)
  arc A202 through (-18.19, 17.7431, -1.2301) (-18.3024, 17.8539, -1.2301) (-18.3899, 17.9852, -1.2301)
  arc A203 through (-17.5907, 19.5622, -1.2301) (-17.725, 19.7897, -1.2301) (-17.858, 20.018, -1.2301)
  arc A204 through (-26.2625, 16.0094, -1.2301) (-26.2826, 16.1143, -1.2301) (-26.316, 16.2157, -1.2301)
  arc A205 through (-34.8615, 15.7886, -1.2301) (-34.8655, 15.3833, -1.2301) (-34.869, 14.978, -1.2301)
  line L37 (-26.1831, 13.1214, -1.2301) -> (-26.2106, 14.6919, -1.2301)
  arc A206 through (-17.77, 17.6295, -1.2301) (-17.8987, 17.6415, -1.2301) (-18.0259, 17.6643, -1.2301)
  line L38 (-26.1881, 12.6149, -1.2301) -> (-25.2881, 12.6149, -1.2301)
  arc A207 through (-34.8437, 11.1569, -1.2301) (-34.8344, 10.8497, -1.2301) (-34.8147, 10.5431, -1.2301)
  arc A208 through (-17.2776, 17.9833, -1.2301) (-17.2435, 17.8878, -1.2301) (-17.2224, 17.7885, -1.2301)
  arc A209 through (-18.3899, 17.9852, -1.2301) (-18.4869, 18.1872, -1.2301) (-18.5686, 18.3959, -1.2301)
  line L39 (-25.0606, 13.0932, -1.2301) -> (-26.1831, 13.1214, -1.2301)
  arc A210 through (-18.7161, 19.997, -1.2301) (-18.675, 20.0685, -1.2301) (-18.5932, 20.0793, -1.2301)
  arc A211 through (-26.6684, 15.2356, -1.2301) (-26.671, 14.7447, -1.2301) (-26.6711, 14.2537, -1.2301)
  arc A212 through (-26.2106, 14.6919, -1.2301) (-26.2199, 15.1509, -1.2301) (-26.2316, 15.6099, -1.2301)
  arc A213 through (-16.8044, 19.9512, -1.2301) (-16.7325, 19.5932, -1.2301) (-16.6982, 19.2296, -1.2301)
  arc A214 through (-28.7891, 17.4399, -1.2301) (-28.7524, 17.4287, -1.2301) (-28.7144, 17.4236, -1.2301)
  arc A215 through (-16.2651, 18.6966, -1.2301) (-16.2036, 19.2867, -1.2301) (-16.2647, 19.8768, -1.2301)
  arc A216 through (-17.1381, 18.8084, -1.2301) (-17.3653, 19.1848, -1.2301) (-17.5907, 19.5622, -1.2301)
  arc A217 through (-18.5932, 20.0793, -1.2301) (-18.4824, 20.0188, -1.2301) (-18.3985, 19.9244, -1.2301)
  line L40 (-34.3881, 11.5989, -1.2301) -> (-34.3381, 13.0329, -1.2301)
  line L41 (-26.6381, 10.1649, -1.2301) -> (-25.2604, 10.1371, -1.2301)
  arc A218 through (-18.2734, 20.7596, -1.2301) (-18.2844, 20.7875, -1.2301) (-18.2881, 20.8172, -1.2301)
  arc A219 through (-28.597, 17.4674, -1.2301) (-28.5376, 17.5539, -1.2301) (-28.5117, 17.6556, -1.2301)
  arc A220 through (-34.7575, 10.2522, -1.2301) (-34.712, 10.1891, -1.2301) (-34.6381, 10.1649, -1.2301)
  arc A221 through (-18.0259, 17.6643, -1.2301) (-18.1125, 17.6943, -1.2301) (-18.19, 17.7431, -1.2301)
  arc A222 through (-18.7381, 19.3117, -1.2301) (-18.7326, 19.6545, -1.2301) (-18.7161, 19.997, -1.2301)
  arc A223 through (-26.6071, 16.2446, -1.2301) (-26.6263, 16.2223, -1.2301) (-26.64, 16.1962, -1.2301)
  line L42 (-25.2881, 10.6149, -1.2301) -> (-26.1881, 10.6149, -1.2301)
  arc A224 through (-34.4237, 10.7094, -1.2301) (-34.4048, 11.1541, -1.2301) (-34.3881, 11.5989, -1.2301)
  line L43 (-23.9104, 11.5871, -1.2301) -> (-23.9381, 13.0649, -1.2301)
  arc A225 through (-26.5523, 16.2806, -1.2301) (-26.5812, 16.2649, -1.2301) (-26.6071, 16.2446, -1.2301)
  arc A226 through (-14.8563, 13.8252, -1.2301) (-14.7751, 13.8375, -1.2301) (-14.6951, 13.8561, -1.2301)
  line L44 (-23.8827, 10.1092, -1.2301) -> (-23.9104, 11.5871, -1.2301)
  line L45 (-23.9381, 13.0649, -1.2301) -> (-25.0606, 13.0932, -1.2301)
  line L46 (-25.2604, 10.1371, -1.2301) -> (-23.8827, 10.1092, -1.2301)
  arc A227 through (-15.3612, 13.8472, -1.2301) (-15.2005, 13.823, -1.2301) (-15.0381, 13.8149, -1.2301)
  arc A228 through (-17.8453, 19.0089, -1.2301) (-17.6462, 18.6686, -1.2301) (-17.4496, 18.3268, -1.2301)
  arc A229 through (-34.6381, 10.1649, -1.2301) (-34.5749, 10.1801, -1.2301) (-34.5253, 10.2222, -1.2301)
  arc A230 through (-34.5253, 10.2222, -1.2301) (-34.4839, 10.2951, -1.2301) (-34.4601, 10.3754, -1.2301)
  arc A231 through (-31.7426, 14.0182, -1.2301) (-31.7392, 14.3916, -1.2301) (-31.7381, 14.7649, -1.2301)
  arc A232 through (-34.4798, 15.987, -1.2301) (-34.6207, 15.9749, -1.2301) (-34.7609, 15.9565, -1.2301)
  line L47 (-26.1881, 11.6149, -1.2301) -> (-26.1881, 12.6149, -1.2301)
  arc A233 through (-14.6951, 13.8561, -1.2301) (-14.63, 13.877, -1.2301) (-14.567, 13.9036, -1.2301)
  arc A234 through (-14.567, 13.9036, -1.2301) (-14.5242, 13.9299, -1.2301) (-14.4881, 13.9649, -1.2301)
  arc A235 through (-31.357, 10.5039, -1.2301) (-31.5603, 10.7809, -1.2301) (-31.7833, 11.0422, -1.2301)
  arc A236 through (-32.9548, 11.5739, -1.2301) (-32.6858, 11.293, -1.2301) (-32.4141, 11.0147, -1.2301)
  arc A237 through (-15.0381, 14.4149, -1.2301) (-15.1292, 14.4124, -1.2301) (-15.22, 14.4047, -1.2301)
  arc A238 through (-15.22, 14.4047, -1.2301) (-15.3011, 14.3923, -1.2301) (-15.3811, 14.3738, -1.2301)
  arc A239 through (-31.7833, 11.0422, -1.2301) (-32.2777, 11.5752, -1.2301) (-32.7772, 12.1034, -1.2301)
  arc A240 through (-14.429, 14.133, -1.2301) (-14.4485, 14.2149, -1.2301) (-14.5007, 14.281, -1.2301)
  arc A241 through (-34.8714, 14.0456, -1.2301) (-34.869, 13.5046, -1.2301) (-34.8647, 12.9636, -1.2301)
  arc A242 through (-6.9381, 12.1281, -1.2301) (-6.5917, 11.9833, -1.2301) (-6.2455, 11.8382, -1.2301)
  arc A243 through (-26.4134, 16.2961, -1.2301) (-26.4487, 16.3001, -1.2301) (-26.4843, 16.2989, -1.2301)
  arc A244 through (-17.6463, 20.9908, -1.2301) (-17.5032, 20.9603, -1.2301) (-17.366, 20.9095, -1.2301)
  arc A245 through (-26.64, 16.1962, -1.2301) (-26.6549, 16.1439, -1.2301) (-26.6603, 16.0898, -1.2301)
  arc A246 through (-26.4843, 16.2989, -1.2301) (-26.519, 16.2923, -1.2301) (-26.5523, 16.2806, -1.2301)
  arc A247 through (-34.8647, 12.9636, -1.2301) (-34.8552, 12.0602, -1.2301) (-34.8437, 11.1569, -1.2301)
  arc A248 through (-26.3857, 20.7556, -1.2301) (-26.4271, 21.2361, -1.2301) (-26.47, 21.7165, -1.2301)
  arc A249 through (-26.3165, 17.3342, -1.2301) (-26.2487, 17.2712, -1.2301) (-26.1765, 17.2132, -1.2301)
  arc A250 through (-26.1066, 18.0675, -1.2301) (-26.1671, 18.3975, -1.2301) (-26.2077, 18.7305, -1.2301)
  arc A251 through (-27.0353, 23.3195, -1.2301) (-27.0644, 23.2499, -1.2301) (-27.0705, 23.1748, -1.2301)
  arc A252 through (-26.9583, 23.3859, -1.2301) (-27.0019, 23.3586, -1.2301) (-27.0353, 23.3195, -1.2301)
  arc A253 through (-8.6951, 25.2624, -1.2301) (-8.715, 25.2467, -1.2301) (-8.7308, 25.2268, -1.2301)
  arc A254 through (-34.3838, 22.8645, -1.2301) (-34.6242, 22.8458, -1.2301) (-34.8645, 22.8254, -1.2301)
  arc A255 through (-14.4158, 17.6709, -1.2301) (-14.4507, 17.6891, -1.2301) (-14.487, 17.7042, -1.2301)
  arc A256 through (-34.8606, 20.8561, -1.2301) (-34.8675, 20.865, -1.2301) (-34.8708, 20.8758, -1.2301)
  arc A257 through (-34.9222, 21.3128, -1.2301) (-34.936, 21.4496, -1.2301) (-34.9491, 21.5864, -1.2301)
  arc A258 through (-26.5493, 22.5394, -1.2301) (-26.5862, 22.8995, -1.2301) (-26.6235, 23.2594, -1.2301)
  arc A259 through (-26.8406, 23.412, -1.2301) (-26.9007, 23.4046, -1.2301) (-26.9583, 23.3859, -1.2301)
  arc A260 through (-14.3457, 17.6223, -1.2301) (-14.3797, 17.648, -1.2301) (-14.4158, 17.6709, -1.2301)
  arc A261 through (-14.487, 17.7042, -1.2301) (-14.5169, 17.7122, -1.2301) (-14.5478, 17.7149, -1.2301)
  arc A262 through (-31.614, 21.0695, -1.2301) (-31.6606, 21.0821, -1.2301) (-31.7088, 21.0849, -1.2301)
  arc A263 through (-34.0564, 22.3783, -1.2301) (-33.8295, 22.3963, -1.2301) (-33.6026, 22.414, -1.2301)
  arc A264 through (-35.2716, 22.7877, -1.2301) (-35.3196, 22.7799, -1.2301) (-35.3662, 22.7661, -1.2301)
  arc A265 through (-12.6471, 17.9005, -1.2301) (-12.7071, 17.8292, -1.2301) (-12.7852, 17.7783, -1.2301)
  line L48 (-34.9491, 21.5864, -1.2301) -> (-35.0151, 22.2961, -1.2301)
  arc A266 through (-31.6375, 22.9095, -1.2301) (-31.7834, 22.9529, -1.2301) (-31.9343, 22.9736, -1.2301)
  arc A267 through (-31.5381, 22.7649, -1.2301) (-31.5654, 22.8526, -1.2301) (-31.6375, 22.9095, -1.2301)
  arc A268 through (-33.9554, 20.4266, -1.2301) (-33.7094, 20.4506, -1.2301) (-33.4634, 20.4735, -1.2301)
  arc A269 through (-32.4413, 20.5642, -1.2301) (-32.2232, 20.5862, -1.2301) (-32.0053, 20.6103, -1.2301)
  arc A270 through (-32.158, 21.0622, -1.2301) (-32.4223, 21.0461, -1.2301) (-32.6863, 21.0273, -1.2301)
  arc A271 through (-13.1962, 17.6034, -1.2301) (-13.4066, 17.5256, -1.2301) (-13.6198, 17.4555, -1.2301)
  arc A272 through (-13.8886, 17.4149, -1.2301) (-13.9461, 17.4177, -1.2301) (-14.003, 17.426, -1.2301)
  arc A273 through (-14.5478, 17.7149, -1.2301) (-14.6641, 17.7467, -1.2301) (-14.7482, 17.8331, -1.2301)
  arc A274 through (-31.9788, 22.5385, -1.2301) (-31.8437, 22.5558, -1.2301) (-31.7105, 22.5839, -1.2301)
  arc A275 through (-12.7852, 17.7783, -1.2301) (-12.9894, 17.6878, -1.2301) (-13.1962, 17.6034, -1.2301)
  arc A276 through (-31.5856, 22.6534, -1.2301) (-31.5505, 22.7043, -1.2301) (-31.5381, 22.7649, -1.2301)
  arc A277 through (-14.7482, 17.8331, -1.2301) (-14.8399, 18.0239, -1.2301) (-14.909, 18.224, -1.2301)
  arc A278 through (-34.8394, 20.8488, -1.2301) (-34.8508, 20.8502, -1.2301) (-34.8606, 20.8561, -1.2301)
  arc A279 through (-12.6556, 18.4924, -1.2301) (-12.6423, 18.2296, -1.2301) (-12.6298, 17.9669, -1.2301)
  arc A280 through (-34.8708, 20.8758, -1.2301) (-34.8835, 20.9774, -1.2301) (-34.8959, 21.0791, -1.2301)
  arc A281 through (-33.1061, 22.4518, -1.2301) (-32.8721, 22.4691, -1.2301) (-32.6381, 22.486, -1.2301)
  arc A282 through (-12.7976, 20.5089, -1.2301) (-12.7727, 20.156, -1.2301) (-12.7453, 19.8033, -1.2301)
  arc A283 through (-33.4634, 20.4735, -1.2301) (-33.2034, 20.4967, -1.2301) (-32.9433, 20.519, -1.2301)
  arc A284 through (-14.909, 18.224, -1.2301) (-14.9875, 18.5459, -1.2301) (-15.0431, 18.8724, -1.2301)
  arc A285 through (-15.0431, 18.8724, -1.2301) (-15.104, 19.3681, -1.2301) (-15.1541, 19.8649, -1.2301)
  arc A286 through (-15.1541, 19.8649, -1.2301) (-15.1809, 20.1569, -1.2301) (-15.2091, 20.4488, -1.2301)
  arc A287 through (-33.289, 20.9767, -1.2301) (-33.5868, 20.95, -1.2301) (-33.8846, 20.924, -1.2301)
  arc A288 through (-34.5704, 20.3568, -1.2301) (-34.4706, 20.3715, -1.2301) (-34.3705, 20.3836, -1.2301)
  arc A289 through (-14.2881, 17.5649, -1.2301) (-14.3156, 17.595, -1.2301) (-14.3457, 17.6223, -1.2301)
  line L49 (-35.0151, 22.2961, -1.2301) -> (-34.3766, 22.3516, -1.2301)
  arc A290 through (-32.6863, 21.0273, -1.2301) (-32.9878, 21.0031, -1.2301) (-33.289, 20.9767, -1.2301)
  arc A291 through (-32.6381, 22.486, -1.2301) (-32.3083, 22.511, -1.2301) (-31.9788, 22.5385, -1.2301)
  arc A292 through (-12.8346, 21.7206, -1.2301) (-12.8505, 21.6835, -1.2301) (-12.8549, 21.6433, -1.2301)
  arc A293 through (-14.003, 17.426, -1.2301) (-14.0619, 17.4401, -1.2301) (-14.1194, 17.459, -1.2301)
  arc A294 through (-32.5253, 22.9763, -1.2301) (-33.1818, 22.9412, -1.2301) (-33.8381, 22.9018, -1.2301)
  arc A295 through (-12.8549, 21.6433, -1.2301) (-12.8441, 21.3809, -1.2301) (-12.8324, 21.1185, -1.2301)
  arc A296 through (-31.5323, 21.0009, -1.2301) (-31.5674, 21.0421, -1.2301) (-31.614, 21.0695, -1.2301)
  arc A297 through (-31.5042, 20.7588, -1.2301) (-31.4913, 20.8198, -1.2301) (-31.4919, 20.8821, -1.2301)
  arc A298 through (-31.6328, 20.6545, -1.2301) (-31.5993, 20.6624, -1.2301) (-31.5683, 20.6772, -1.2301)
  arc A299 through (-33.8846, 20.924, -1.2301) (-34.1371, 20.903, -1.2301) (-34.3897, 20.883, -1.2301)
  arc A300 through (-12.6298, 17.9669, -1.2301) (-12.6334, 17.9324, -1.2301) (-12.6471, 17.9005, -1.2301)
  arc A301 through (-34.3705, 20.3836, -1.2301) (-34.163, 20.4055, -1.2301) (-33.9554, 20.4266, -1.2301)
  arc A302 through (-32.0053, 20.6103, -1.2301) (-31.819, 20.6321, -1.2301) (-31.6328, 20.6545, -1.2301)
  arc A303 through (-34.3897, 20.883, -1.2301) (-34.6146, 20.8658, -1.2301) (-34.8394, 20.8488, -1.2301)
  arc A304 through (-32.9433, 20.519, -1.2301) (-32.6922, 20.5409, -1.2301) (-32.4413, 20.5642, -1.2301)
  arc A305 through (-31.7105, 22.5839, -1.2301) (-31.6435, 22.6105, -1.2301) (-31.5856, 22.6534, -1.2301)
  arc A306 through (-31.7088, 21.0849, -1.2301) (-31.9334, 21.0741, -1.2301) (-32.158, 21.0622, -1.2301)
  arc A307 through (-33.6026, 22.414, -1.2301) (-33.3543, 22.433, -1.2301) (-33.1061, 22.4518, -1.2301)
  arc A308 through (-12.8324, 21.1185, -1.2301) (-12.8166, 20.8136, -1.2301) (-12.7976, 20.5089, -1.2301)
  arc A309 through (-13.6198, 17.4555, -1.2301) (-13.7527, 17.4251, -1.2301) (-13.8886, 17.4149, -1.2301)
  arc A310 through (-34.8959, 21.0791, -1.2301) (-34.9096, 21.1959, -1.2301) (-34.9222, 21.3128, -1.2301)
  arc A311 through (-12.7453, 19.8033, -1.2301) (-12.7178, 19.4511, -1.2301) (-12.6923, 19.0988, -1.2301)
  arc A312 through (-12.165, 21.7687, -1.2301) (-12.2931, 21.8001, -1.2301) (-12.4238, 21.8172, -1.2301)
  arc A313 through (-13.2681, 17.0324, -1.2301) (-13.125, 17.0866, -1.2301) (-12.9841, 17.1463, -1.2301)
  arc A314 through (-10.2263, 19.3922, -1.2301) (-10.2156, 19.5814, -1.2301) (-10.2048, 19.7705, -1.2301)
  arc A315 through (-12.1655, 21.5421, -1.2301) (-12.1437, 21.5517, -1.2301) (-12.1248, 21.5663, -1.2301)
  arc A316 through (-14.7713, 17.2517, -1.2301) (-14.5777, 17.1373, -1.2301) (-14.3729, 17.0444, -1.2301)
  arc A317 through (-15.3353, 21.4899, -1.2301) (-15.3656, 21.5413, -1.2301) (-15.4118, 21.5791, -1.2301)
  arc A318 through (-12.6923, 19.0988, -1.2301) (-12.6726, 18.7957, -1.2301) (-12.6556, 18.4924, -1.2301)
  arc A319 through (-10.1995, 19.7961, -1.2301) (-10.1929, 19.8048, -1.2301) (-10.1824, 19.8082, -1.2301)
  arc A320 through (-31.4919, 20.8821, -1.2301) (-31.5058, 20.9437, -1.2301) (-31.5323, 21.0009, -1.2301)
  arc A321 through (-10.7095, 17.3606, -1.2301) (-10.6885, 17.286, -1.2301) (-10.6492, 17.2192, -1.2301)
  arc A322 through (-31.5683, 20.6772, -1.2301) (-31.529, 20.7123, -1.2301) (-31.5042, 20.7588, -1.2301)
  line L50 (-10.6881, 20.4089, -1.2301) -> (-11.2131, 20.4369, -1.2301)
  arc A323 through (-12.4238, 21.8172, -1.2301) (-12.5619, 21.8202, -1.2301) (-12.6996, 21.8085, -1.2301)
  arc A324 through (-31.9343, 22.9736, -1.2301) (-32.2297, 22.983, -1.2301) (-32.5253, 22.9763, -1.2301)
  arc A325 through (-13.7339, 16.9373, -1.2301) (-13.6211, 16.9466, -1.2301) (-13.5095, 16.965, -1.2301)
  arc A326 through (-10.4257, 17.2184, -1.2301) (-10.3836, 17.2853, -1.2301) (-10.3586, 17.3604, -1.2301)
  line L51 (-34.9027, 20.3031, -1.2301) -> (-34.5704, 20.3568, -1.2301)
  arc A327 through (-14.1194, 17.459, -1.2301) (-14.1711, 17.481, -1.2301) (-14.2206, 17.5074, -1.2301)
  arc A328 through (-14.2206, 17.5074, -1.2301) (-14.2569, 17.5333, -1.2301) (-14.2881, 17.5649, -1.2301)
  arc A329 through (-34.3766, 22.3516, -1.2301) (-34.2165, 22.3653, -1.2301) (-34.0564, 22.3783, -1.2301)
  arc A330 through (-15.6364, 19.7058, -1.2301) (-15.5522, 19.0074, -1.2301) (-15.4613, 18.3098, -1.2301)
  arc A331 through (-12.0881, 21.6649, -1.2301) (-12.1094, 21.7295, -1.2301) (-12.165, 21.7687, -1.2301)
  arc A332 through (-10.7338, 17.6731, -1.2301) (-10.7269, 17.5164, -1.2301) (-10.7095, 17.3606, -1.2301)
  arc A333 through (-13.965, 16.9448, -1.2301) (-13.8496, 16.9367, -1.2301) (-13.7339, 16.9373, -1.2301)
  arc A334 through (-12.2131, 21.5399, -1.2301) (-12.1892, 21.5381, -1.2301) (-12.1655, 21.5421, -1.2301)
  arc A335 through (-12.1248, 21.5663, -1.2301) (-12.1088, 21.5864, -1.2301) (-12.0976, 21.6095, -1.2301)
  arc A336 through (-12.9841, 17.1463, -1.2301) (-12.7229, 17.2721, -1.2301) (-12.4694, 17.4127, -1.2301)
  arc A337 through (-12.4694, 17.4127, -1.2301) (-12.3489, 17.5123, -1.2301) (-12.2649, 17.6441, -1.2301)
  arc A338 through (-10.618, 21.7517, -1.2301) (-10.6363, 21.7263, -1.2301) (-10.6457, 21.6963, -1.2301)
  line L52 (-10.6881, 21.0453, -1.2301) -> (-10.6881, 20.4089, -1.2301)
  arc A339 through (-12.1979, 17.9918, -1.2301) (-12.2159, 18.4177, -1.2301) (-12.2434, 18.8431, -1.2301)
  arc A340 through (-10.683, 21.2941, -1.2301) (-10.6868, 21.1697, -1.2301) (-10.6881, 21.0453, -1.2301)
  arc A341 through (-11.5176, 20.4473, -1.2301) (-11.5852, 20.4428, -1.2301) (-11.651, 20.4271, -1.2301)
  arc A342 through (-11.2131, 20.4369, -1.2301) (-11.3653, 20.4436, -1.2301) (-11.5176, 20.4473, -1.2301)
  arc A343 through (-11.651, 20.4271, -1.2301) (-11.6888, 20.4054, -1.2301) (-11.7148, 20.3704, -1.2301)
  arc A344 through (-11.7118, 20.161, -1.2301) (-11.6811, 20.1192, -1.2301) (-11.64, 20.0875, -1.2301)
  arc A345 through (-15.4118, 21.5791, -1.2301) (-15.4733, 21.6035, -1.2301) (-15.539, 21.6112, -1.2301)
  arc A346 through (-15.539, 21.6112, -1.2301) (-15.6053, 21.6016, -1.2301) (-15.6669, 21.5755, -1.2301)
  arc A347 through (-11.7381, 20.2649, -1.2301) (-11.7315, 20.2113, -1.2301) (-11.7118, 20.161, -1.2301)
  line L53 (-10.7381, 19.8952, -1.2301) -> (-10.7381, 18.53, -1.2301)
  arc A348 through (-15.1062, 17.5331, -1.2301) (-14.9466, 17.3832, -1.2301) (-14.7713, 17.2517, -1.2301)
  arc A349 through (-12.3163, 19.998, -1.2301) (-12.3312, 20.4225, -1.2301) (-12.333, 20.8473, -1.2301)
  arc A350 through (-15.7447, 21.4839, -1.2301) (-15.7882, 21.3133, -1.2301) (-15.7911, 21.1373, -1.2301)
  arc A351 through (-12.333, 20.8473, -1.2301) (-12.3258, 21.1559, -1.2301) (-12.3112, 21.4643, -1.2301)
  arc A352 through (-15.2629, 20.961, -1.2301) (-15.2875, 21.1788, -1.2301) (-15.3127, 21.3965, -1.2301)
  arc A353 through (-10.6457, 21.6963, -1.2301) (-10.6576, 21.6059, -1.2301) (-10.6675, 21.5153, -1.2301)
  arc A354 through (-10.6675, 21.5153, -1.2301) (-10.6769, 21.4048, -1.2301) (-10.683, 21.2941, -1.2301)
  arc A355 through (-15.6669, 21.5755, -1.2301) (-15.7136, 21.5363, -1.2301) (-15.7447, 21.4839, -1.2301)
  arc A356 through (-15.2091, 20.4488, -1.2301) (-15.2351, 20.705, -1.2301) (-15.2629, 20.961, -1.2301)
  arc A357 through (-15.3252, 17.8518, -1.2301) (-15.2284, 17.6837, -1.2301) (-15.1062, 17.5331, -1.2301)
  arc A358 through (-12.3112, 21.4643, -1.2301) (-12.2794, 21.5244, -1.2301) (-12.2131, 21.5399, -1.2301)
  arc A359 through (-12.0976, 21.6095, -1.2301) (-12.0905, 21.6368, -1.2301) (-12.0881, 21.6649, -1.2301)
  arc A360 through (-11.4994, 20.0325, -1.2301) (-11.3692, 20.0043, -1.2301) (-11.2381, 19.98, -1.2301)
  line L54 (-11.2381, 19.98, -1.2301) -> (-10.7381, 19.8952, -1.2301)
  arc A361 through (-10.2048, 19.7705, -1.2301) (-10.2031, 19.7835, -1.2301) (-10.1995, 19.7961, -1.2301)
  arc A362 through (-14.3729, 17.0444, -1.2301) (-14.1722, 16.9811, -1.2301) (-13.965, 16.9448, -1.2301)
  arc A363 through (-13.5095, 16.965, -1.2301) (-13.3876, 16.9945, -1.2301) (-13.2681, 17.0324, -1.2301)
  arc A364 through (-10.2493, 18.9655, -1.2301) (-10.238, 19.1789, -1.2301) (-10.2263, 19.3922, -1.2301)
  arc A365 through (-10.6492, 17.2192, -1.2301) (-10.5999, 17.1792, -1.2301) (-10.5381, 17.1649, -1.2301)
  arc A366 through (-15.7911, 21.1373, -1.2301) (-15.7164, 20.4212, -1.2301) (-15.6364, 19.7058, -1.2301)
  arc A367 through (-15.3127, 21.3965, -1.2301) (-15.3212, 21.4439, -1.2301) (-15.3353, 21.4899, -1.2301)
  arc A368 through (-11.7148, 20.3704, -1.2301) (-11.7322, 20.3189, -1.2301) (-11.7381, 20.2649, -1.2301)
  arc A369 through (-10.3586, 17.3604, -1.2301) (-10.3331, 17.5137, -1.2301) (-10.3182, 17.6684, -1.2301)
  arc A370 through (-12.2434, 18.8431, -1.2301) (-12.2835, 19.4203, -1.2301) (-12.3163, 19.998, -1.2301)
  arc A371 through (-10.3182, 17.6684, -1.2301) (-10.2952, 18.0666, -1.2301) (-10.2745, 18.4649, -1.2301)
  arc A372 through (-10.2745, 18.4649, -1.2301) (-10.2621, 18.7152, -1.2301) (-10.2493, 18.9655, -1.2301)
  arc A373 through (-12.2649, 17.6441, -1.2301) (-12.2121, 17.8142, -1.2301) (-12.1979, 17.9918, -1.2301)
  arc A374 through (-12.6996, 21.8085, -1.2301) (-12.7769, 21.7797, -1.2301) (-12.8346, 21.7206, -1.2301)
  arc A375 through (-22.3982, 19.6701, -1.2301) (-22.3722, 19.2078, -1.2301) (-22.349, 18.7453, -1.2301)
  arc A376 through (-22.2736, 17.6744, -1.2301) (-22.2515, 17.4645, -1.2301) (-22.2279, 17.2548, -1.2301)
  arc A377 through (-11.64, 20.0875, -1.2301) (-11.5717, 20.0549, -1.2301) (-11.4994, 20.0325, -1.2301)
  arc A378 through (-15.4613, 18.3098, -1.2301) (-15.4109, 18.0755, -1.2301) (-15.3252, 17.8518, -1.2301)
  arc A379 through (-10.7381, 18.53, -1.2301) (-10.737, 18.1016, -1.2301) (-10.7338, 17.6731, -1.2301)
  arc A380 through (-10.5381, 17.1649, -1.2301) (-10.4759, 17.179, -1.2301) (-10.4257, 17.2184, -1.2301)
  arc A381 through (-9.137, 20.1984, -1.2301) (-9.3228, 20.2284, -1.2301) (-9.509, 20.2552, -1.2301)
  arc A382 through (-22.0105, 17.1325, -1.2301) (-21.9765, 17.1387, -1.2301) (-21.9434, 17.1491, -1.2301)
  arc A383 through (-22.0812, 17.1323, -1.2301) (-22.0458, 17.1303, -1.2301) (-22.0105, 17.1325, -1.2301)
  line L55 (-21.8515, 18.7457, -1.2301) -> (-21.9177, 20.2817, -1.2301)
  arc A384 through (-10.523, 21.7926, -1.2301) (-10.5519, 21.7859, -1.2301) (-10.58, 21.7765, -1.2301)
  arc A385 through (-22.349, 18.7453, -1.2301) (-22.3339, 18.4585, -1.2301) (-22.3158, 18.1719, -1.2301)
  arc A386 through (-23.6741, 19.3577, -1.2301) (-23.6803, 19.6082, -1.2301) (-23.6839, 19.8589, -1.2301)
  arc A387 through (-10.4574, 21.7984, -1.2301) (-10.4903, 21.797, -1.2301) (-10.523, 21.7926, -1.2301)
  arc A388 through (-23.8802, 17.1321, -1.2301) (-23.8452, 17.1302, -1.2301) (-23.8103, 17.1324, -1.2301)
  arc A389 through (-23.6867, 20.294, -1.2301) (-23.6806, 20.3088, -1.2301) (-23.6659, 20.3149, -1.2301)
  arc A390 through (-9.108, 19.7825, -1.2301) (-9.0252, 19.7863, -1.2301) (-8.9436, 19.8011, -1.2301)
  arc A391 through (-22.1903, 17.1771, -1.2301) (-22.1691, 17.16, -1.2301) (-22.1447, 17.1477, -1.2301)
  arc A392 through (-21.9434, 17.1491, -1.2301) (-21.8903, 17.1855, -1.2301) (-21.8595, 17.242, -1.2301)
  arc A393 through (-21.8595, 17.242, -1.2301) (-21.8358, 17.351, -1.2301) (-21.8236, 17.462, -1.2301)
  arc A394 through (-10.3164, 21.7401, -1.2301) (-10.3493, 21.7742, -1.2301) (-10.393, 21.7923, -1.2301)
  arc A395 through (-21.8236, 17.462, -1.2301) (-21.8165, 17.6641, -1.2301) (-21.8185, 17.8663, -1.2301)
  arc A396 through (-23.7434, 17.1491, -1.2301) (-23.6902, 17.1856, -1.2301) (-23.6594, 17.2424, -1.2301)
  arc A397 through (-22.3158, 18.1719, -1.2301) (-22.2967, 17.923, -1.2301) (-22.2736, 17.6744, -1.2301)
  arc A398 through (-10.2648, 21.619, -1.2301) (-10.2858, 21.6816, -1.2301) (-10.3164, 21.7401, -1.2301)
  arc A399 through (-21.8185, 17.8663, -1.2301) (-21.8338, 18.306, -1.2301) (-21.8515, 18.7457, -1.2301)
  arc A400 through (-10.209, 21.0541, -1.2301) (-10.2181, 21.2318, -1.2301) (-10.2305, 21.4094, -1.2301)
  arc A401 through (-22.1447, 17.1477, -1.2301) (-22.1134, 17.138, -1.2301) (-22.0812, 17.1323, -1.2301)
  arc A402 through (-22.9246, 20.5568, -1.2301) (-22.8679, 20.5458, -1.2301) (-22.8153, 20.5219, -1.2301)
  line L56 (-21.9177, 20.2817, -1.2301) -> (-21.5279, 20.4378, -1.2301)
  arc A403 through (-9.9932, 19.809, -1.2301) (-9.8829, 19.8082, -1.2301) (-9.7727, 19.8059, -1.2301)
  arc A404 through (-23.6839, 19.8589, -1.2301) (-23.6855, 20.0764, -1.2301) (-23.6867, 20.294, -1.2301)
  arc A405 through (-23.6659, 20.3149, -1.2301) (-23.648, 20.3164, -1.2301) (-23.6307, 20.3208, -1.2301)
  arc A406 through (-23.6594, 17.2424, -1.2301) (-23.6358, 17.3525, -1.2301) (-23.6237, 17.4644, -1.2301)
  arc A407 through (-23.8103, 17.1324, -1.2301) (-23.7763, 17.1387, -1.2301) (-23.7434, 17.1491, -1.2301)
  arc A408 through (-9.7727, 19.8059, -1.2301) (-9.6429, 19.8016, -1.2301) (-9.5131, 19.7961, -1.2301)
  arc A409 through (-23.6522, 18.7623, -1.2301) (-23.6641, 19.06, -1.2301) (-23.6741, 19.3577, -1.2301)